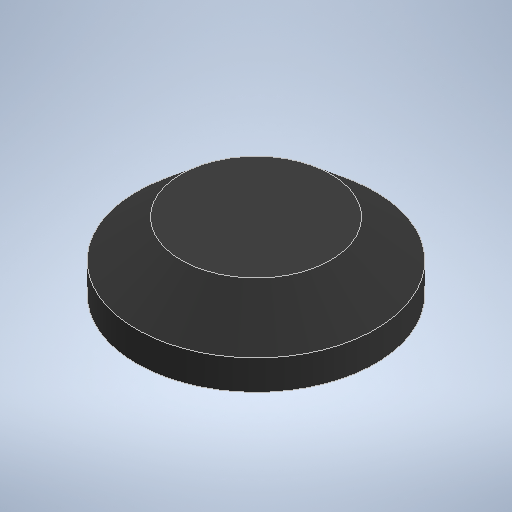
# Autodesk Inventor part: Pe_nivelador
Saved by Autodesk Inventor 2025.2 (Build 292293000, 293)
## iProperties
Created: 2025-04-08
Part Number: Pe_nivelador
Material: Rubber
Document SubType Name: Modeling
Designer: kenne
Density: 0.93 g/cm^3
Appearance: Rubber - Black
Author: kenne
Autodesk Inventor part; units mm, degrees
ref_plane "YZ Plane" through (0, 0, 0) normal (1, 0, 0) x (0, 1, 0)
ref_plane "XZ Plane" through (0, 0, 0) normal (0, 1, 0) x (-1, 0, 0)
ref_plane "XY Plane" through (0, 0, 0) normal (0, 0, 1) x (1, 0, 0)
sketch "base_sketch" plane through (0, 0, 0) normal (0, 0, 1) x (1, 0, 0)
  line L0 (-100, -25) -> (0, -25)
  line L1 (-100, 0) -> (0, 0)
  line L2 (0, 0) -> (-100, 0) construction
  line L3 (-100, 0) -> (-100, -25)
  line L4 (0, 0) -> (0, 100) construction
  line L5 (-100, 0) -> (-62.5264, 31.4441)
  line L6 (-62.5264, 31.4441) -> (0, 31.4441)
  line L7 (0, 31.4441) -> (0, -25)
  point P0 (-50, -25)
  dimension "d0" = 100
  dimension "d1" = 25
  dimension "d2" = 100
  dimension "d3" = 100
  dimension "d4" = 130
  dimension "d5" = 62.5264
  constraints: 16 end point, 2 horizontal, 2 point on line, 2 vertical, 2 vertical alignment, 1 coincident, 1 midpoint, 1 parallel, 1 perpendicular
  measures "d0" distance of L0.start L0.end
  measures "d1" vertical distance of point (0, 0) point (-50, -25)
  measures "d2" distance of L1.end L2.end
  measures "d3" distance of L1.end L4.end
  measures "d4" angle of L3 L5
  measures "d5" distance of L5.end L6.end
revolve "base_Revolution" add sketch "base_sketch" angle 360 about axis through (0, 0, 0) along (0, 1, 0)
body "Solid1"
